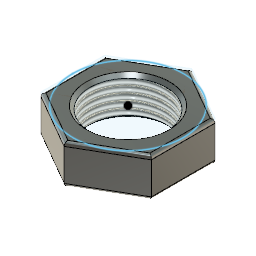
Semana3_Desafio6 v1 (Autodesk Fusion 360 design; units mm, degrees)
Autodesk Fusion 360 part; units mm, degrees
sketch "Sketch1" plane through (0, 0, 0) normal (0, 0, 1) x (1, 0, 0)
  line L0 (50, 28.8675) -> (0, 57.735)
  line L1 (0, 57.735) -> (-50, 28.8675)
  line L2 (-50, 28.8675) -> (-50, -28.8675)
  line L3 (-50, -28.8675) -> (0, -57.735)
  line L4 (0, -57.735) -> (50, -28.8675)
  line L5 (50, -28.8675) -> (50, 28.8675)
extrude "Extrude1" add sketch "Sketch1" along normal blind 35
sketch "Sketch2" plane through (0, 0, 35) normal (0, 0, 1) x (-1, 0, 0)
  line L0 (-50, 28.8675) -> (-50, -28.8675)
  line L1 (-50, -28.8675) -> (0, -57.735)
  line L2 (0, -57.735) -> (50, -28.8675)
  line L3 (50, -28.8675) -> (50, 28.8675)
  line L4 (50, 28.8675) -> (0, 57.735)
  line L5 (0, 57.735) -> (-50, 28.8675)
  circle A0 centre (0, 0) radius 50
  constraint coincident A0.centre origin
hole "Hole1" at (0, 0, 35) direction (0, 0, -1) diameter 75 depth 35 tip angle 180
thread "Thread1" "ISO Metric profile 75.0 M75x6 6H" major diameter 75.6205 minor diameter 68.9048 pitch 6 angle 60 resizes the face on face at (3.7338, -37.3137, 23.3333)
chamfer "Chamfer1" distance 3 angle 45 1 edges at (-32.1209, 12.4585, 35)
fillet "Fillet2" radius 3 6 edges at (-25, -43.3013, 35) (25, -43.3013, 35) (-50, 0, 35) (-25, 43.3013, 35) (25, 43.3013, 35) (50, 0, 35)
fillet "Fillet3" radius 3 6 edges at (25, -43.3013, 0) (-25, -43.3013, 0) (50, 0, 0) (25, 43.3013, 0) (-25, 43.3013, 0) (-50, 0, 0)
chamfer "Chamfer2" distance 3 angle 45 1 edges at (-32.1209, -12.4585, 0)
